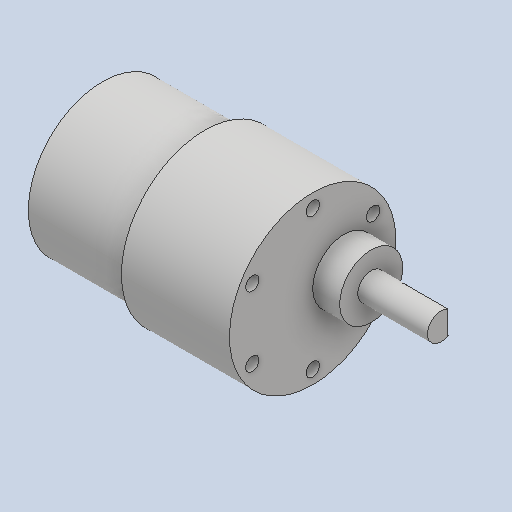
# Autodesk Inventor part: DCMotor
Saved by Autodesk Inventor 2023 (Build 270158000, 158)
## iProperties
Created: 2022-08-31
Part Number: DCMotor
Material: Generic
Document SubType Name: Modeling
Designer: Nathann
Density: 1 g/cm^3
Appearance: Default
Author: Nathann
Autodesk Inventor part; units mm, degrees
ref_plane "YZ Plane" through (0, 0, 0) normal (1, 0, 0) x (0, 1, 0)
ref_plane "XZ Plane" through (0, 0, 0) normal (0, 1, 0) x (-1, 0, 0)
ref_plane "XY Plane" through (0, 0, 0) normal (0, 0, 1) x (1, 0, 0)
sketch "Sketch1" plane through (0, 0, 0) normal (1, 0, 0) x (0, 1, 0)
  circle A0 centre (0, 0) radius 16.5
  dimension "d0" = 33
  constraints: 1 centre point, 1 coincident
  measures "d0" diameter of A0
extrude "Extrusion1" add sketch "Sketch1" along normal blind 22.7
sketch "Sketch2" plane through (22.7, 0, 0) normal (1, 0, 0) x (0, 0, -1)
  circle A0 centre (0, 0) radius 18.5
  dimension "d3" = 37
  constraints: 1 centre point, 1 coincident
  measures "d3" diameter of A0
extrude "Extrusion2" add sketch "Sketch2" along normal blind 24
sketch "Sketch3" plane through (46.7, 0, 0) normal (1, 0, 0) x (0, 0, -1)
  circle A0 centre (0, 7) radius 7
  point P0 (0, 0)
  dimension "d6" = 14
  dimension "d7" = 7
  constraints: 1 centre point
  measures "d6" diameter of A0
  measures "d7" distance of point (0, 0) A0.centre
extrude "Extrusion3" add sketch "Sketch3" along normal blind 6
sketch "Sketch4" plane through (52.7, 7, 0) normal (1, 0, 0) x (0, 0, -1)
  circle A0 centre (0, 0) radius 3
  point P0 (0, -7)
  dimension "d10" = 6
  constraints: 1 centre point
  measures "d10" diameter of A0
extrude "Extrusion4" add sketch "Sketch4" along normal blind 15.5
sketch "Sketch5" plane through (46.7, 0, 0) normal (1, 0, 0) x (0, 0, -1)
  circle A0 centre (-15.5, 0) radius 1.5
  circle A1 centre (0, 7) radius 7 projected
  circle A2 centre (-7.75, -13.4234) radius 1.5
  circle A3 centre (7.75, -13.4234) radius 1.5
  circle A4 centre (15.5, 0) radius 1.5
  circle A5 centre (7.75, 13.4234) radius 1.5
  circle A6 centre (-7.75, 13.4234) radius 1.5
  point P0 (0, 0)
  dimension "d13" = 3
  dimension "d14" = 15.5
  dimension "d17" = 360
  constraints: 6 centre point, 1 vertical alignment, 13 other
  measures "d13" diameter of A0
  measures "d14" horizontal distance of point (0, 7) A0.centre
extrude "Extrusion5" cut sketch "Sketch5" against normal blind 10 contours A0 | A2 | A3 | A4 | A5 | A6
sketch "Sketch6" plane through (68.2, 7, 0) normal (1, 0, 0) x (0, 0, -1)
  line L0 (-3.2783, 3.4497) -> (2.5487, 3.4497)
  line L1 (2.5487, 3.4497) -> (2.5487, 1.5658)
  line L2 (2.5487, 1.5658) -> (-3.2783, 1.5658)
  line L3 (-3.2783, 1.5658) -> (-3.2783, 3.4497)
  point P0 (0, -7)
  constraints: 8 end point, 2 parallel, 1 horizontal, 1 perpendicular
extrude "Extrusion6" cut sketch "Sketch6" against normal blind 10
body "Solid1"
